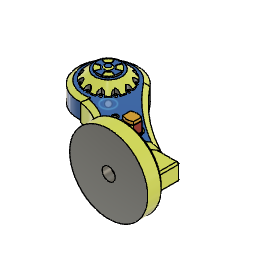
Jaw v2 (Autodesk Fusion 360 design; units mm, degrees)
Autodesk Fusion 360 part; units mm, degrees
note: some values were not read from the file. Set by a fixed rule: which sketch regions a step uses.
sketch "Sketch1" plane through (0, 0, 20) normal (0, 0, 1) x (1, 0, 0)
  line L0 (-77.5, 37) -> (77.5, 37)
  line L1 (77.5, 37) -> (77.5, 87)
  line L2 (77.5, 87) -> (-77.5, 87)
  line L3 (-77.5, 87) -> (-77.5, 37)
  line L4 (-77.5, 87) -> (32.5, 87)
  line L5 (-77.5, 87) -> (-77.5, 48)
  arc A0 (-77.5, 48) -> (32.5, 87) centre (-68.6761, 197.7402) ccw
  dimension "d1" = 110
  dimension "d2" = 39
  dimension "d3" = 150
  constraint coincident L2.end L3.start
  measures "d1" distance of L2.end L4.end
  measures "d2" distance of L2.end L5.end
  measures "d3" radius of A0
sketch "Sketch2" plane through (0, 0, 49.5) normal (0, 0, 1) x (1, 0, 0)
  circle A0 centre (-160.5089, 159.5313) radius 31
  circle A1 centre (-160.5089, 159.5313) radius 50
  circle A2 centre (-160.5089, 159.5313) radius 50
  line L0 (-160.5089, 159.5313) -> (-160.5089, 209.5313)
  arc A3 (-167.6812, 209.0142) -> (-160.5089, 200.5313) centre (-158.6873, 209.3451) ccw
  arc A4 (-160.5089, 200.5313) -> (-153.3365, 209.0142) centre (-162.3304, 209.3451) ccw
  dimension "d4" = 9
  dimension "d5" = 9
  constraint coincident A0.centre A1.centre
  constraint vertical L0
  constraint coincident L0 A3.end
  constraint coincident A1 A3.start
  constraint symmetric L0 A3.start A4.end
  constraint symmetric L0 A3.end A4.start
  constraint symmetric L0 A3 A4
  measures "d4" distance of L0.end A3.end
  measures "d5" radius of A3
sketch "Sketch3" plane through (0, 0, 27.5) normal (0, 0, 1) x (1, 0, 0)
  line L0 (-145.4858, 103.7293) -> (-145.1519, 99.3765)
  arc A0 (-72.5215, 58.5044) -> (-145.1519, 99.3765) centre (-172.177, -33.6165) ccw
  arc A1 (-72.5215, 58.5044) -> (13.4424, 85.2327) centre (-68.6761, 197.7402) ccw
  arc A2 (-115.3255, 195.5593) -> (13.4424, 85.2327) centre (237.072, 476.5514) ccw
  arc A3 (-115.3255, 195.5593) -> (-145.4858, 103.7293) centre (-160.5089, 159.5313) ccw
  circle A4 centre (-160.5089, 159.5313) radius 50
  dimension "d6" = 100
  constraint concentric A3 A4
  measures "d6" diameter of A4
sketch "Sketch4" plane through (0, 0, 27.5) normal (0, 0, 1) x (1, 0, 0)
  arc A0 (-167.6812, 209.0142) -> (-153.3365, 209.0142) centre (-160.5089, 159.5313) ccw
  arc A1 (-167.6812, 209.0142) -> (-160.5089, 200.5313) centre (-158.6873, 209.3451) ccw
  arc A2 (-160.5089, 200.5313) -> (-153.3365, 209.0142) centre (-162.3304, 209.3451) ccw
  line L0 (-145.4858, 103.7293) -> (-145.1519, 99.3765)
  arc A3 (-72.5215, 58.5044) -> (-145.1519, 99.3765) centre (-172.177, -33.6165) ccw
  arc A4 (-72.5215, 58.5044) -> (13.4424, 85.2327) centre (-68.6761, 197.7402) ccw
  arc A5 (-115.3255, 195.5593) -> (13.4424, 85.2327) centre (237.072, 476.5514) ccw
  arc A6 (-115.3255, 195.5593) -> (-145.4858, 103.7293) centre (-160.5089, 159.5313) ccw
  line L1 (-160.5089, 200.5313) -> (-160.5089, 217.3225)
  circle A7 centre (-160.5089, 206.9289) radius 3
  circle A8 centre (-160.5089, 206.9289) radius 1.6
  dimension "d7" = 6
  dimension "d8" = 1.4
  constraint coincident A1.end A2.start
  constraint vertical L1
  constraint coincident L1 A7.centre
  measures "d7" diameter of A7
sketch "Sketch5" plane through (0, 0, 49.5) normal (0, 0, 1) x (1, 0, 0)
  circle A0 centre (-160.5089, 159.5313) radius 31
  circle A1 centre (-160.5089, 159.5313) radius 13
  circle A2 centre (-160.5089, 159.5313) radius 25
  dimension "d9" = 26
  dimension "d10" = 50
  constraint concentric A0 A1
  constraint concentric A1 A2
  measures "d9" diameter of A1
  measures "d10" diameter of A2
sketch "Sketch6" plane through (0, 0, 52.5) normal (0, 0, 1) x (1, 0, 0)
  circle A0 centre (-160.5089, 159.5313) radius 25
  circle A1 centre (-160.5089, 159.5313) radius 13
  line L0 (-164.9551, 171.7473) -> (-169.0594, 183.0236)
  line L1 (-156.0626, 171.7473) -> (-151.9584, 183.0236)
  line L2 (-172.7249, 163.9776) -> (-184.0012, 168.0818)
  line L3 (-172.7249, 155.0851) -> (-184.0012, 150.9808)
  line L4 (-164.9551, 147.3153) -> (-169.0594, 136.039)
  line L5 (-156.0626, 147.3153) -> (-151.9584, 136.039)
  line L6 (-148.2928, 155.0851) -> (-137.0165, 150.9808)
  line L7 (-148.2928, 163.9776) -> (-137.0165, 168.0818)
  dimension "d11" = 26
  constraint concentric A0 A1
  constraint coincident A0 L0.end
  constraint coincident A1 L0.start
  measures "d11" diameter of A1
sketch "Sketch7" plane through (0, 0, 53.5) normal (0, 0, 1) x (1, 0, 0)
  line L0 (-156.0626, 171.7473) -> (-151.9584, 183.0236)
  arc A0 (-151.9584, 183.0236) -> (-169.0594, 183.0236) centre (-160.5089, 159.5313) ccw
  line L1 (-169.0594, 183.0236) -> (-164.9551, 171.7473)
  arc A1 (-164.9551, 171.7473) -> (-172.7249, 163.9776) centre (-160.5089, 159.5313) ccw
  line L2 (-172.7249, 163.9776) -> (-184.0012, 168.0818)
  arc A2 (-184.0012, 168.0818) -> (-184.0012, 150.9808) centre (-160.5089, 159.5313) ccw
  line L3 (-184.0012, 150.9808) -> (-172.7249, 155.0851)
  arc A3 (-172.7249, 155.0851) -> (-164.9551, 147.3153) centre (-160.5089, 159.5313) ccw
  line L4 (-164.9551, 147.3153) -> (-169.0594, 136.039)
  arc A4 (-169.0594, 136.039) -> (-151.9584, 136.039) centre (-160.5089, 159.5313) ccw
  line L5 (-151.9584, 136.039) -> (-156.0626, 147.3153)
  arc A5 (-156.0626, 147.3153) -> (-148.2928, 155.0851) centre (-160.5089, 159.5313) ccw
  line L6 (-148.2928, 155.0851) -> (-137.0165, 150.9808)
  arc A6 (-137.0165, 150.9808) -> (-137.0165, 168.0818) centre (-160.5089, 159.5313) ccw
  line L7 (-137.0165, 168.0818) -> (-148.2928, 163.9776)
  arc A7 (-148.2928, 163.9776) -> (-156.0626, 171.7473) centre (-160.5089, 159.5313) ccw
  circle A8 centre (-160.5089, 159.5313) radius 9.5
  dimension "d12" = 19
  constraint concentric A0 A8
  measures "d12" diameter of A8
sketch "Sketch8" plane through (0, 0, 0) normal (0, 1, 0) x (1, 0, 0)
  circle A0 centre (0, 0) radius 90
  dimension "d13" = 180
  constraint coincident A0.centre origin
  measures "d13" diameter of A0
sketch "Sketch9" plane through (0, 0, 0) normal (0, 0, 1) x (1, 0, 0)
  line L0 (90, 0) -> (-90, 0)
  line L1 (1.7286, 0) -> (-148.2714, 0)
  line L2 (-148.2714, 0) -> (-160.5089, 159.5313)
  circle A0 centre (-160.5089, 159.5313) radius 68.5
  arc A1 (-77.5, 48) -> (-164.6394, 91.156) centre (-172.177, -33.6165) ccw
  arc A2 (-106.9508, 202.2371) -> (32.5, 87) centre (237.072, 476.5514) ccw
  arc A3 (-77.5, 48) -> (32.5, 87) centre (-68.6761, 197.7402) ccw
  arc A4 (-77.5, 48) -> (32.5, 87) centre (-68.6761, 197.7402) ccw
  point P0 (-77.5, 48)
  point P1 (32.5, 87)
  dimension "d14" = 150
  dimension "d15" = 160
  dimension "d16" = 137
  dimension "d17" = 125
  dimension "d18" = 440
  constraint coincident L0 L1.start
  constraint coincident L2.end A0.centre
  constraint coincident P0 A1.start
  constraint coincident A0 A1.end
  constraint coincident P1 A2.end
  constraint coincident A0 A2.start
  constraint tangent A0 A2
  constraint tangent A0 A1
  measures "d14" distance of L1.start L1.end
  measures "d15" distance of L1.end L2.end
  measures "d16" diameter of A0
  measures "d17" radius of A1
  measures "d18" radius of A2
sketch "Sketch10" plane through (0, 0, 20) normal (0, 0, 1) x (1, 0, 0)
  line L0 (-77.5, 48) -> (-77.5, 37)
  line L1 (-77.5, 37) -> (77.5, 37)
  line L2 (77.5, 37) -> (77.5, 87)
  line L3 (77.5, 87) -> (32.5, 87)
  arc A0 (-106.9508, 202.2371) -> (32.5, 87) centre (237.072, 476.5514) ccw
  arc A1 (-106.9508, 202.2371) -> (-155.2697, 91.232) centre (-160.5089, 159.5313) ccw
  line L4 (-155.2697, 91.232) -> (-155.1924, 90.2242)
  arc A2 (-77.5, 48) -> (-155.1924, 90.2242) centre (-172.177, -33.6165) ccw
  circle A3 centre (-160.5089, 159.5313) radius 68.5
  arc A4 (-77.5, 48) -> (-164.6394, 91.156) centre (-172.177, -33.6165) ccw
  arc A5 (-106.9508, 202.2371) -> (32.5, 87) centre (237.072, 476.5514) ccw
  arc A6 (-77.5, 48) -> (32.5, 87) centre (-68.6761, 197.7402) ccw
sketch "Sketch11" plane through (0, 37, 0) normal (0, 1, 0) x (-1, 0, 0)
  circle A0 centre (0, 0) radius 84
  line L0 (-77.5, -20) -> (77.5, -20)
  line L1 (77.5, -20) -> (77.5, 20)
  line L2 (77.5, 20) -> (-77.5, 20)
  line L3 (-77.5, 20) -> (-77.5, -20)
  line L4 (-77.5, -20) -> (77.5, 20) construction
  line L5 (77.5, -20) -> (-77.5, 20) construction
  dimension "d19" = 155
  dimension "d20" = 40
  constraint perpendicular L0 L1
  constraint parallel L0 L2
  constraint parallel L1 L3
  constraint horizontal L0
  constraint coincident L4 A0.centre
  constraint coincident L5 A0.centre
  constraint coincident A0.centre origin
  measures "d19" distance of L1.end L2.end
  measures "d20" distance of L0.end L1.end
sketch "Sketch12" plane through (0, 0, 27.5) normal (0, 0, 1) x (1, 0, 0)
  line L0 (-18.1736, 94.9006) -> (-18.1736, 75.9006)
  arc A0 (-45.1736, 75.9006) -> (-18.1736, 75.9006) centre (-31.6736, 99.2833) ccw
  line L1 (-45.1736, 75.9006) -> (-45.1736, 94.9006)
  arc A1 (-18.1736, 94.9006) -> (-45.1736, 94.9006) centre (-31.6736, 71.5179) ccw
  circle A2 centre (-201.5563, 183.2301) radius 3
  circle A3 centre (-201.5563, 135.8326) radius 3
  circle A4 centre (-160.5089, 112.1338) radius 3
  circle A5 centre (-119.4614, 135.8326) radius 3
  circle A6 centre (-119.4614, 183.2301) radius 3
  circle A7 centre (-160.5089, 206.9289) radius 3
  arc A8 (-141.9789, 205.971) -> (-153.3365, 209.0142) centre (-160.5089, 159.5313) ccw
  arc A9 (-141.9789, 205.971) -> (-140.0089, 195.0384) centre (-134.0245, 201.7605) ccw
  arc A10 (-140.0089, 195.0384) -> (-129.5559, 198.7986) centre (-137.1795, 203.5821) ccw
  arc A11 (-121.2416, 190.4842) -> (-129.5559, 198.7986) centre (-160.5089, 159.5313) ccw
  arc A12 (-121.2416, 190.4842) -> (-125.0018, 180.0313) centre (-116.4581, 182.8607) ccw
  arc A13 (-125.0018, 180.0313) -> (-114.0692, 178.0613) centre (-118.2797, 186.0157) ccw
  arc A14 (-111.026, 166.7037) -> (-114.0692, 178.0613) centre (-160.5089, 159.5313) ccw
  arc A15 (-111.026, 166.7037) -> (-119.5089, 159.5313) centre (-110.6951, 157.7098) ccw
  arc A16 (-119.5089, 159.5313) -> (-111.026, 152.3589) centre (-110.6951, 161.3529) ccw
  arc A17 (-114.0692, 141.0013) -> (-111.026, 152.3589) centre (-160.5089, 159.5313) ccw
  arc A18 (-114.0692, 141.0013) -> (-125.0018, 139.0313) centre (-118.2797, 133.047) ccw
  arc A19 (-125.0018, 139.0313) -> (-121.2416, 128.5784) centre (-116.4581, 136.202) ccw
  arc A20 (-129.5559, 120.2641) -> (-121.2416, 128.5784) centre (-160.5089, 159.5313) ccw
  arc A21 (-129.5559, 120.2641) -> (-140.0089, 124.0243) centre (-137.1795, 115.4806) ccw
  arc A22 (-140.0089, 124.0243) -> (-141.9789, 113.0917) centre (-134.0245, 117.3021) ccw
  arc A23 (-153.3365, 110.0484) -> (-141.9789, 113.0917) centre (-160.5089, 159.5313) ccw
  arc A24 (-153.3365, 110.0484) -> (-160.5089, 118.5313) centre (-162.3304, 109.7176) ccw
  arc A25 (-160.5089, 118.5313) -> (-167.6812, 110.0484) centre (-158.6873, 109.7176) ccw
  arc A26 (-179.0388, 113.0917) -> (-167.6812, 110.0484) centre (-160.5089, 159.5313) ccw
  arc A27 (-179.0388, 113.0917) -> (-181.0089, 124.0243) centre (-186.9932, 117.3021) ccw
  arc A28 (-181.0089, 124.0243) -> (-191.4618, 120.2641) centre (-183.8382, 115.4806) ccw
  arc A29 (-199.7761, 128.5784) -> (-191.4618, 120.2641) centre (-160.5089, 159.5313) ccw
  arc A30 (-199.7761, 128.5784) -> (-196.0159, 139.0313) centre (-204.5596, 136.202) ccw
  arc A31 (-196.0159, 139.0313) -> (-206.9485, 141.0013) centre (-202.7381, 133.047) ccw
  arc A32 (-209.9917, 152.3589) -> (-206.9485, 141.0013) centre (-160.5089, 159.5313) ccw
  arc A33 (-209.9917, 152.3589) -> (-201.5089, 159.5313) centre (-210.3226, 161.3529) ccw
  arc A34 (-201.5089, 159.5313) -> (-209.9917, 166.7037) centre (-210.3226, 157.7098) ccw
  arc A35 (-206.9485, 178.0613) -> (-209.9917, 166.7037) centre (-160.5089, 159.5313) ccw
  arc A36 (-206.9485, 178.0613) -> (-196.0159, 180.0313) centre (-202.7381, 186.0157) ccw
  arc A37 (-196.0159, 180.0313) -> (-199.7761, 190.4842) centre (-204.5596, 182.8607) ccw
  arc A38 (-191.4618, 198.7986) -> (-199.7761, 190.4842) centre (-160.5089, 159.5313) ccw
  arc A39 (-191.4618, 198.7986) -> (-181.0089, 195.0384) centre (-183.8382, 203.5821) ccw
  arc A40 (-181.0089, 195.0384) -> (-179.0388, 205.971) centre (-186.9932, 201.7605) ccw
  arc A41 (-167.6812, 209.0142) -> (-179.0388, 205.971) centre (-160.5089, 159.5313) ccw
  arc A42 (-167.6812, 209.0142) -> (-160.5089, 200.5313) centre (-158.6873, 209.3451) ccw
  arc A43 (-160.5089, 200.5313) -> (-153.3365, 209.0142) centre (-162.3304, 209.3451) ccw
  line L2 (-145.4858, 103.7293) -> (-145.1519, 99.3765)
  arc A44 (-72.5215, 58.5044) -> (-145.1519, 99.3765) centre (-172.177, -33.6165) ccw
  arc A45 (-72.5215, 58.5044) -> (13.4424, 85.2327) centre (-68.6761, 197.7402) ccw
  arc A46 (-115.3255, 195.5593) -> (13.4424, 85.2327) centre (237.072, 476.5514) ccw
  arc A47 (-115.3255, 195.5593) -> (-145.4858, 103.7293) centre (-160.5089, 159.5313) ccw
  circle A48 centre (-136.8101, 200.5788) radius 3
  circle A49 centre (-113.1113, 159.5313) radius 3
  circle A50 centre (-136.8101, 118.4838) radius 3
  circle A51 centre (-184.2076, 118.4838) radius 3
  circle A52 centre (-207.9064, 159.5313) radius 3
  circle A53 centre (-184.2076, 200.5788) radius 3
  line L3 (-18.1736, 94.9006) -> (-45.1736, 75.9006)
  line L4 (-45.1736, 94.9006) -> (-18.1736, 75.9006)
  circle A54 centre (-31.6736, 85.4006) radius 19.9859
  circle A55 centre (-31.6736, 85.4006) radius 17.4107
  circle A56 centre (-80, 95) radius 6.5
  circle A57 centre (-80, 95) radius 3.5
  dimension "d21" = 13
  dimension "d22" = 7
  constraint coincident L0.start A1.start
  constraint coincident A0.start L1.start
  constraint coincident L1.end A1.end
  constraint coincident L0.end A0.end
  constraint midpoint L4 A54.centre
  constraint concentric A54 A55
  constraint concentric A56 A57
  measures "d21" diameter of A56
  measures "d22" diameter of A57
sketch "Sketch13" plane through (0, 0, 27.5) normal (0, 0, 1) x (1, 0, 0)
  circle A0 centre (-201.5563, 183.2301) radius 3
  circle A1 centre (-201.5563, 135.8326) radius 3
  circle A2 centre (-160.5089, 112.1338) radius 3
  circle A3 centre (-119.4614, 135.8326) radius 3
  circle A4 centre (-119.4614, 183.2301) radius 3
  circle A5 centre (-160.5089, 206.9289) radius 3
  arc A6 (-141.9789, 205.971) -> (-153.3365, 209.0142) centre (-160.5089, 159.5313) ccw
  arc A7 (-141.9789, 205.971) -> (-140.0089, 195.0384) centre (-134.0245, 201.7605) ccw
  arc A8 (-140.0089, 195.0384) -> (-129.5559, 198.7986) centre (-137.1795, 203.5821) ccw
  arc A9 (-121.2416, 190.4842) -> (-129.5559, 198.7986) centre (-160.5089, 159.5313) ccw
  arc A10 (-121.2416, 190.4842) -> (-125.0018, 180.0313) centre (-116.4581, 182.8607) ccw
  arc A11 (-125.0018, 180.0313) -> (-114.0692, 178.0613) centre (-118.2797, 186.0157) ccw
  arc A12 (-111.026, 166.7037) -> (-114.0692, 178.0613) centre (-160.5089, 159.5313) ccw
  arc A13 (-111.026, 166.7037) -> (-119.5089, 159.5313) centre (-110.6951, 157.7098) ccw
  arc A14 (-119.5089, 159.5313) -> (-111.026, 152.3589) centre (-110.6951, 161.3529) ccw
  arc A15 (-114.0692, 141.0013) -> (-111.026, 152.3589) centre (-160.5089, 159.5313) ccw
  arc A16 (-114.0692, 141.0013) -> (-125.0018, 139.0313) centre (-118.2797, 133.047) ccw
  arc A17 (-125.0018, 139.0313) -> (-121.2416, 128.5784) centre (-116.4581, 136.202) ccw
  arc A18 (-129.5559, 120.2641) -> (-121.2416, 128.5784) centre (-160.5089, 159.5313) ccw
  arc A19 (-129.5559, 120.2641) -> (-140.0089, 124.0243) centre (-137.1795, 115.4806) ccw
  arc A20 (-140.0089, 124.0243) -> (-141.9789, 113.0917) centre (-134.0245, 117.3021) ccw
  arc A21 (-153.3365, 110.0484) -> (-141.9789, 113.0917) centre (-160.5089, 159.5313) ccw
  arc A22 (-153.3365, 110.0484) -> (-160.5089, 118.5313) centre (-162.3304, 109.7176) ccw
  arc A23 (-160.5089, 118.5313) -> (-167.6812, 110.0484) centre (-158.6873, 109.7176) ccw
  arc A24 (-179.0388, 113.0917) -> (-167.6812, 110.0484) centre (-160.5089, 159.5313) ccw
  arc A25 (-179.0388, 113.0917) -> (-181.0089, 124.0243) centre (-186.9932, 117.3021) ccw
  arc A26 (-181.0089, 124.0243) -> (-191.4618, 120.2641) centre (-183.8382, 115.4806) ccw
  arc A27 (-199.7761, 128.5784) -> (-191.4618, 120.2641) centre (-160.5089, 159.5313) ccw
  arc A28 (-199.7761, 128.5784) -> (-196.0159, 139.0313) centre (-204.5596, 136.202) ccw
  arc A29 (-196.0159, 139.0313) -> (-206.9485, 141.0013) centre (-202.7381, 133.047) ccw
  arc A30 (-209.9917, 152.3589) -> (-206.9485, 141.0013) centre (-160.5089, 159.5313) ccw
  arc A31 (-209.9917, 152.3589) -> (-201.5089, 159.5313) centre (-210.3226, 161.3529) ccw
  arc A32 (-201.5089, 159.5313) -> (-209.9917, 166.7037) centre (-210.3226, 157.7098) ccw
  arc A33 (-206.9485, 178.0613) -> (-209.9917, 166.7037) centre (-160.5089, 159.5313) ccw
  arc A34 (-206.9485, 178.0613) -> (-196.0159, 180.0313) centre (-202.7381, 186.0157) ccw
  arc A35 (-196.0159, 180.0313) -> (-199.7761, 190.4842) centre (-204.5596, 182.8607) ccw
  arc A36 (-191.4618, 198.7986) -> (-199.7761, 190.4842) centre (-160.5089, 159.5313) ccw
  arc A37 (-191.4618, 198.7986) -> (-181.0089, 195.0384) centre (-183.8382, 203.5821) ccw
  arc A38 (-181.0089, 195.0384) -> (-179.0388, 205.971) centre (-186.9932, 201.7605) ccw
  arc A39 (-167.6812, 209.0142) -> (-179.0388, 205.971) centre (-160.5089, 159.5313) ccw
  arc A40 (-167.6812, 209.0142) -> (-160.5089, 200.5313) centre (-158.6873, 209.3451) ccw
  arc A41 (-160.5089, 200.5313) -> (-153.3365, 209.0142) centre (-162.3304, 209.3451) ccw
  line L0 (-145.4858, 103.7293) -> (-145.1519, 99.3765)
  arc A42 (-72.5215, 58.5044) -> (-145.1519, 99.3765) centre (-172.177, -33.6165) ccw
  arc A43 (-72.5215, 58.5044) -> (13.4424, 85.2327) centre (-68.6761, 197.7402) ccw
  arc A44 (-115.3255, 195.5593) -> (13.4424, 85.2327) centre (237.072, 476.5514) ccw
  arc A45 (-115.3255, 195.5593) -> (-145.4858, 103.7293) centre (-160.5089, 159.5313) ccw
  circle A46 centre (-136.8101, 200.5788) radius 3
  circle A47 centre (-113.1113, 159.5313) radius 3
  circle A48 centre (-136.8101, 118.4838) radius 3
  circle A49 centre (-184.2076, 118.4838) radius 3
  circle A50 centre (-207.9064, 159.5313) radius 3
  circle A51 centre (-184.2076, 200.5788) radius 3
  line L1 (-45.1736, 94.9006) -> (-18.1736, 94.9006)
  line L2 (-18.1736, 94.9006) -> (-18.1736, 75.9006)
  line L3 (-18.1736, 75.9006) -> (-45.1736, 75.9006)
  line L4 (-45.1736, 75.9006) -> (-45.1736, 94.9006)
  arc A52 (-18.1736, 94.9006) -> (-45.1736, 94.9006) centre (-31.6736, 71.5179) ccw
  arc A53 (-45.1736, 75.9006) -> (-18.1736, 75.9006) centre (-31.6736, 99.2833) ccw
  dimension "d23" = 27
  dimension "d24" = 19
  dimension "d25" = 27
  dimension "d26" = 27
  constraint horizontal L1
  constraint vertical L2
  constraint horizontal L3
  constraint vertical L4
  measures "d23" distance of L1.start L1.end
  measures "d24" distance of L1.start L3.end
  measures "d25" radius of A52
  measures "d26" radius of A53
sketch "Sketch14" plane through (0, 0, 28.5) normal (0, 0, 1) x (1, 0, 0)
  arc A0 (-18.1736, 94.9006) -> (-45.1736, 94.9006) centre (-31.6736, 71.5179) ccw
  line L0 (-45.1736, 94.9006) -> (-45.1736, 75.9006)
  arc A1 (-45.1736, 75.9006) -> (-18.1736, 75.9006) centre (-31.6736, 99.2833) ccw
  line L1 (-18.1736, 75.9006) -> (-18.1736, 94.9006)
sketch "Sketch15" plane through (0, 0, 0) normal (0, -1, 0) x (1, 0, 0)
  circle A0 centre (0, 0) radius 90
  circle A1 centre (0, 0) radius 15
  dimension "d27" = 30
  constraint coincident A0.centre A1.centre
  measures "d27" diameter of A1
sketch "Sketch16" plane through (0, 0, 49.5) normal (0, 0, 1) x (1, 0, 0)
  line L0 (-18.1736, 75.9006) -> (-18.1736, 94.9006)
  arc A0 (-18.1736, 94.9006) -> (-45.1736, 94.9006) centre (-31.6736, 71.5179) ccw
  line L1 (-45.1736, 94.9006) -> (-45.1736, 75.9006)
  arc A1 (-45.1736, 75.9006) -> (-18.1736, 75.9006) centre (-31.6736, 99.2833) ccw
  arc A2 (-44.1736, 76.4853) -> (-19.1736, 76.4853) centre (-31.6736, 99.2833) ccw
  line L2 (-19.1736, 76.4853) -> (-19.1736, 94.316)
  arc A3 (-19.1736, 94.316) -> (-44.1736, 94.316) centre (-31.6736, 71.5179) ccw
  line L3 (-44.1736, 94.316) -> (-44.1736, 76.4853)
  dimension "d28" = 1
extrude "Extrude1" add sketch "Sketch8" along normal blind 37
chamfer "Chamfer1" distance 6 angle 45 1 edges at (-83.9095, 37, 32.5454)
extrude "Extrude2" add sketch "Sketch11" along normal blind 50 contours L0 L1 L2 L3
extrude "Extrude3" cut sketch "Sketch1" against normal blind 100 contours L2 L3 L4 L5 A0
extrude "Extrude4" add sketch "Sketch9" along normal mid plane 40 contours L2 A0 A1 A2 A3 A4 | A0
extrude "Extrude5" add sketch "Sketch10" along normal blind 7.5 draft -55 contours A0 L4 A2 A3 A4 A5 A6 | A1 A3
extrude "Extrude6" add sketch "Sketch3" along normal blind 3 contours A4
extrude "Extrude7" add 1 faces at (-177.9053, 167.497, 30.5) along direction (0, 0, 1) blind 19 draft -45
extrude "Extrude8" cut sketch "Sketch2" against normal up to surface (22 mm away) contours A1 A2 L0 A4 | A1 A2 L0 A3
extrude "Extrude9" add sketch "Sketch4" along normal blind 3 contours L1 A7 A8 | L1 A7 A8
pattern_circular "C-Pattern1" count 12 over 360 about axis through (-160.5089, 159.5313, 49.5) along (0, 0, -1) of "Extrude8", "Extrude9"
extrude "Extrude10" add sketch "Sketch5" along normal blind 3 contours A1 | A2
extrude "Extrude11" add sketch "Sketch6" along normal blind 1 contours A0 A1 L6 L7 | A0 A1 L0 L1 | A1 | A0 A1 L4 L5 | A0 A1 L2 L3
extrude "Extrude12" add sketch "Sketch7" along normal blind 3 draft -45 contours A8
extrude "Extrude13" add sketch "Sketch13" along normal blind 1 contours L1 A52 | L1 L2 L3 L4 | L3 A53
extrude "Extrude14" add sketch "Sketch14" along normal blind 21
extrude "Extrude15" add sketch "Sketch16" along normal blind 7 contours A2 L2 A3 L3
extrude "Extrude16" cut sketch "Sketch12" against normal blind 0.5 contours A54 | A56
extrude "Extrude17" cut sketch "Sketch15" against normal blind 20 contours A1
fillet "Fillet1" radius 4 9 edges at (-223.3166, 186.8706, -20) (-43.2117, 137.3744, -20) (55, 87, -20) (55, 87, 20) (77.5, 87, 0) (77.5, 62, 20) (77.5, 62, -20) (-77.5, 42.5, -20) (-77.5, 42.5, 20)
move_body "Move1" bodies 1 to x (1, 0, 0) y (0, 1, 0) z (0, 0, 1) at (-400, 0, 0)
sketch "sketch 3049" plane through (25.5794, -35.1239, -20) normal (0, 0, -1) x (-1, 0, 0)
  circle A0 centre (586.0883, 194.6552) radius 15
extrude "Extrude18" cut sketch "sketch 3049" against normal blind 20
